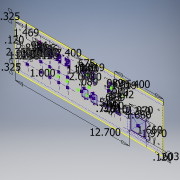
# Autodesk Inventor part: PDU_chassis
Saved by Autodesk Inventor 2017 (Build 210142000, 142)
## iProperties
Created: 2017-02-13
Part Number: PDU_chassis
Material: Generic
Document SubType Name: Modeling
Designer: Zara
Density: 1 g/cm^3
Appearance: Default
Author: Zara
Autodesk Inventor part; units mm, degrees
ref_plane "YZ Plane" through (0, 0, 0) normal (1, 0, 0) x (0, 1, 0)
ref_plane "XZ Plane" through (0, 0, 0) normal (0, 1, 0) x (-1, 0, 0)
ref_plane "XY Plane" through (0, 0, 0) normal (0, 0, 1) x (1, 0, 0)
sketch "Sketch1" plane through (0, 0, 0) normal (0, 0, 1) x (1, 0, 0)
  line L0 (-209.423, -66.294) -> (209.423, -66.294)
  line L1 (209.423, -66.294) -> (209.423, 66.294)
  line L2 (209.423, 66.294) -> (-209.423, 66.294)
  line L3 (-209.423, 66.294) -> (-209.423, -66.294)
  line L4 (-209.423, -66.294) -> (209.423, 66.294) construction
  line L5 (209.423, -66.294) -> (-209.423, 66.294) construction
  point P0 (0, 0)
  dimension "d0" = 418.846
  dimension "d1" = 132.588
  constraints: 12 end point, 2 midpoint, 2 parallel, 1 horizontal, 1 perpendicular
  measures "d0" distance of L1.end L2.end
  measures "d1" distance of L0.end L1.end
extrude "pdu" add sketch "Sketch1" along normal blind 1.651
sketch "dsub9 sketch" plane through (0, 0, 1.651) normal (0, 0, 1) x (1, 0, 0)
  line L0 (206.375, 58.039) -> (-206.375, 58.039) construction
  line L1 (-206.375, 58.039) -> (-206.375, -58.039) construction
  line L2 (-206.375, -58.039) -> (206.375, -58.039) construction
  line L3 (206.375, -58.039) -> (206.375, 58.039) construction
  line L4 (209.423, 66.294) -> (-209.423, 66.294) construction
  line L5 (-209.423, -66.294) -> (209.423, -66.294) construction
  line L6 (-209.423, 66.294) -> (-209.423, -66.294) construction
  line L7 (209.423, -66.294) -> (209.423, 66.294) construction
  arc A0 (-131.445, 36.9951) -> (-133.3231, 38.571) centre (-133.0452, 36.9951) ccw
  arc A1 (-133.3231, 19.3918) -> (-131.445, 20.9677) centre (-133.0452, 20.9677) ccw
  arc A2 (-142.621, 22.374) -> (-141.2987, 20.7981) centre (-141.0208, 22.374) ccw
  arc A3 (-141.2987, 37.1647) -> (-142.621, 35.5888) centre (-141.0208, 35.5888) ccw
  line L8 (-131.445, 36.9951) -> (-131.445, 20.9677)
  line L9 (-142.621, 35.5888) -> (-142.621, 22.374)
  line L10 (-141.2987, 37.1647) -> (-133.3231, 38.571)
  line L11 (-133.3231, 19.3918) -> (-141.2987, 20.7981)
  line L12 (-131.445, 28.9814) -> (-142.621, 28.9814) construction
  line L13 (-137.033, 41.4814) -> (-137.033, 16.4814) construction
  arc A4 (-117.221, 22.374) -> (-115.8987, 20.7981) centre (-115.6208, 22.374) ccw
  arc A5 (-107.9231, 19.3918) -> (-106.045, 20.9677) centre (-107.6452, 20.9677) ccw
  line L14 (-106.045, 28.9814) -> (-117.221, 28.9814) construction
  arc A6 (-115.8987, 37.1647) -> (-117.221, 35.5888) centre (-115.6208, 35.5888) ccw
  line L15 (-115.8987, 37.1647) -> (-107.9231, 38.571)
  line L16 (-106.045, 36.9951) -> (-106.045, 20.9677)
  arc A7 (-106.045, 36.9951) -> (-107.9231, 38.571) centre (-107.6452, 36.9951) ccw
  line L17 (-111.633, 41.4814) -> (-111.633, 16.4814) construction
  line L18 (-107.9231, 19.3918) -> (-115.8987, 20.7981)
  line L19 (-117.221, 35.5888) -> (-117.221, 22.374)
  arc A8 (-91.821, 22.374) -> (-90.4987, 20.7981) centre (-90.2208, 22.374) ccw
  arc A9 (-82.5231, 19.3918) -> (-80.645, 20.9677) centre (-82.2452, 20.9677) ccw
  line L20 (-80.645, 28.9814) -> (-91.821, 28.9814) construction
  arc A10 (-90.4987, 37.1647) -> (-91.821, 35.5888) centre (-90.2208, 35.5888) ccw
  line L21 (-90.4987, 37.1647) -> (-82.5231, 38.571)
  line L22 (-80.645, 36.9951) -> (-80.645, 20.9677)
  arc A11 (-80.645, 36.9951) -> (-82.5231, 38.571) centre (-82.2452, 36.9951) ccw
  line L23 (-86.233, 41.4814) -> (-86.233, 16.4814) construction
  line L24 (-82.5231, 19.3918) -> (-90.4987, 20.7981)
  line L25 (-91.821, 35.5888) -> (-91.821, 22.374)
  arc A12 (-66.421, 22.374) -> (-65.0987, 20.7981) centre (-64.8208, 22.374) ccw
  arc A13 (-57.1231, 19.3918) -> (-55.245, 20.9677) centre (-56.8452, 20.9677) ccw
  line L26 (-55.245, 28.9814) -> (-66.421, 28.9814) construction
  arc A14 (-65.0987, 37.1647) -> (-66.421, 35.5888) centre (-64.8208, 35.5888) ccw
  line L27 (-65.0987, 37.1647) -> (-57.1231, 38.571)
  line L28 (-55.245, 36.9951) -> (-55.245, 20.9677)
  arc A15 (-55.245, 36.9951) -> (-57.1231, 38.571) centre (-56.8452, 36.9951) ccw
  line L29 (-60.833, 41.4814) -> (-60.833, 16.4814) construction
  line L30 (-57.1231, 19.3918) -> (-65.0987, 20.7981)
  line L31 (-66.421, 35.5888) -> (-66.421, 22.374)
  line L32 (-131.445, 32.3846) -> (-131.445, 46.6583) construction
  line L33 (-131.445, 25.0932) -> (-131.445, 19.1695) construction
  line L34 (-135.9942, 38.1) -> (-131.189, 38.9473) construction
  line L35 (-133.9716, 19.5062) -> (-131.2614, 19.0283) construction
  line L36 (-131.445, 24.4508) -> (-131.445, 17.8692) construction
  point P0 (0, 0)
  point P1 (-137.033, 28.9814)
  point P2 (-111.633, 28.9814)
  point P3 (-86.233, 28.9814)
  point P4 (-60.833, 28.9814)
  point P5 (-131.445, 19.0607)
  point P6 (-131.445, 38.9021)
  dimension "d24" = 38.1
  dimension "d13" = 8.255
  dimension "d14" = 8.255
  dimension "d15" = 3.048
  dimension "d16" = 3.048
  dimension "d381" = 3.2004
  dimension "d386" = 3.2004
  dimension "d391" = 3.2004
  dimension "d396" = 3.2004
  dimension "d397" = 16.0274
  dimension "d399" = 11.176
  dimension "d401" = 25
  dimension "d402" = 37.3126
  dimension "d403" = 72.39
  dimension "d406" = 25.4
  dimension "d420" = 100
  dimension "d425" = 19.8415
  constraints: 66 end point, 32 point on circle, 16 centre point, 10 point on line, 8 coincident, 8 tangent, 5 vertical, 4 midpoint, 3 horizontal, 2 parallel, 2 perpendicular, 1 collinear, 86 other
  measures "d13" distance between parallel lines of L4 L0
  measures "d14" distance between parallel lines of L5 L2
  measures "d15" distance between parallel lines of L6 L1
  measures "d16" distance between parallel lines of L7 L3
  measures "d381" diameter of A0
  measures "d386" diameter of A1
  measures "d391" diameter of A2
  measures "d396" diameter of A3
  measures "d397" distance of A1.centre A0.centre
  measures "d399" distance between parallel lines of L9 L8
  measures "d401" distance of L13.start L13.end
  measures "d402" distance between parallel lines of L4 L12
  measures "d403" distance between parallel lines of L13 L6
  measures "d406" distance of A2.centre A4.centre
  measures "d420" angle of L11 L8
  measures "d425" distance of point (-131.445, 38.902) point (-131.445, 19.061)
sketch "CAT7 sketch" plane through (0, 0, 1.651) normal (0, 0, 1) x (1, 0, 0)
  line L0 (-21.463, 40.4114) -> (-4.318, 40.4114)
  line L1 (-4.318, 40.4114) -> (-4.318, 17.5514)
  line L2 (-4.318, 17.5514) -> (-21.463, 17.5514)
  line L3 (-21.463, 17.5514) -> (-21.463, 40.4114)
  line L4 (-29.3489, 28.9814) -> (14.0188, 28.9814) construction
  circle A0 centre (-12.8905, 43.4848) radius 1.1303
  circle A1 centre (-12.8905, 14.478) radius 1.1303
  line L5 (-12.8905, 43.4848) -> (-12.8905, 14.478) construction
  line L6 (-209.423, -66.294) -> (209.423, -66.294) construction
  line L7 (-209.423, 66.294) -> (-209.423, -66.294) construction
  line L8 (32.9446, 29.4386) -> (89.0123, 29.4386) construction
  line L9 (55.7784, 40.4114) -> (71.6026, 40.4114)
  line L10 (72.263, 39.751) -> (72.263, 18.2118)
  line L11 (71.6026, 17.5514) -> (55.7784, 17.5514)
  line L12 (55.118, 18.2118) -> (55.118, 39.751)
  circle A2 centre (63.6905, 43.942) radius 1.1303
  circle A3 centre (63.6905, 14.9352) radius 1.1303
  line L13 (63.6905, 43.942) -> (63.6905, 14.9352) construction
  line L14 (209.423, 66.294) -> (-209.423, 66.294) projected
  line L15 (-209.423, -66.294) -> (209.423, -66.294) projected
  line L16 (209.423, -66.294) -> (209.423, 66.294) projected
  line L17 (209.423, 66.294) -> (-209.423, 66.294) projected
  line L18 (-209.423, 66.294) -> (-209.423, -66.294) projected
  line L19 (3.937, 40.4114) -> (21.082, 40.4114)
  line L20 (21.082, 40.4114) -> (21.082, 17.5514)
  line L21 (21.082, 17.5514) -> (3.937, 17.5514)
  line L22 (3.937, 17.5514) -> (3.937, 40.4114)
  line L23 (12.5095, 43.4848) -> (12.5095, 14.478) construction
  circle A4 centre (12.5095, 43.4848) radius 1.1303
  circle A5 centre (12.5095, 14.478) radius 1.1303
  line L24 (-21.463, -10.3886) -> (-4.318, -10.3886)
  line L25 (-4.318, -10.3886) -> (-4.318, -33.2486)
  line L26 (-4.318, -33.2486) -> (-21.463, -33.2486)
  line L27 (-21.463, -33.2486) -> (-21.463, -10.3886)
  line L28 (-12.8905, -7.3152) -> (-12.8905, -36.322) construction
  circle A6 centre (-12.8905, -7.3152) radius 1.1303
  circle A7 centre (-12.8905, -36.322) radius 1.1303
  line L29 (3.937, -10.3886) -> (21.082, -10.3886)
  line L30 (21.082, -10.3886) -> (21.082, -33.2486)
  line L31 (21.082, -33.2486) -> (3.937, -33.2486)
  line L32 (3.937, -33.2486) -> (3.937, -10.3886)
  line L33 (12.5095, -7.3152) -> (12.5095, -36.322) construction
  circle A8 centre (12.5095, -7.3152) radius 1.1303
  circle A9 centre (12.5095, -36.322) radius 1.1303
  line L34 (-12.8905, -21.8186) -> (115.0098, -21.8186) construction
  arc A10 (72.263, 39.751) -> (71.6026, 40.4114) centre (71.6026, 39.751) ccw
  arc A11 (55.7784, 40.4114) -> (55.118, 39.751) centre (55.7784, 39.751) ccw
  arc A12 (55.118, 18.2118) -> (55.7784, 17.5514) centre (55.7784, 18.2118) ccw
  arc A13 (71.6026, 17.5514) -> (72.263, 18.2118) centre (71.6026, 18.2118) ccw
  point P0 (-21.463, 28.9814)
  point P1 (-12.8905, 40.4114)
  point P2 (-12.8905, 28.9814)
  point P3 (55.118, 40.4114)
  point P4 (72.263, 17.5514)
  point P5 (72.263, 40.4114)
  point P6 (55.118, 17.5514)
  point P7 (55.118, 28.9814)
  point P8 (63.6905, 40.4114)
  point P9 (63.6905, 29.4386)
  point P10 (98.2853, 29.4386)
  point P11 (12.5095, 40.4114)
  point P12 (3.937, 28.9814)
  point P13 (-3.9489, 28.9814)
  point P14 (12.5095, 28.9814)
  point P15 (-12.8905, -10.3886)
  point P16 (-21.463, -21.8186)
  point P17 (-29.3489, -21.8186)
  point P18 (12.5095, -10.3886)
  point P19 (3.937, -21.8186)
  point P20 (-3.9489, -21.8186)
  point P21 (12.5095, -21.8186)
  dimension "d56" = 47.0408
  dimension "d47" = 22.86
  dimension "d49" = 2.2606
  dimension "d50" = 2.2606
  dimension "d51" = 29.0068
  dimension "d146" = 22.86
  dimension "d147" = 17.145
  dimension "d148" = 2.2606
  dimension "d149" = 2.2606
  dimension "d150" = 29.0068
  dimension "d152" = 25.8826
  dimension "d236" = 25.4
  dimension "d239" = 50.8
  dimension "d243" = 137.16
  dimension "d244" = 187.96
  dimension "d245" = 17.145
  dimension "d246" = 25.8826
  dimension "d421" = 0.6604
  constraints: 56 end point, 15 point on line, 14 centre point, 8 point on circle, 8 tangent, 6 midpoint, 5 horizontal, 4 parallel, 4 vertical, 3 equal radius, 2 collinear, 2 perpendicular, 49 other
  measures "d47" distance of L0.end L1.end
  measures "d49" diameter of A0
  measures "d50" diameter of A1
  measures "d51" distance of L5.end L5.start
  measures "d146" distance of point (72.263, 40.411) point (72.263, 17.551)
  measures "d147" distance of point (72.263, 17.551) point (55.118, 17.551)
  measures "d148" diameter of A2
  measures "d149" diameter of A3
  measures "d150" distance of L13.end L13.start
  measures "d152" distance between parallel lines of L14 L9
  measures "d236" distance of L0.start L19.start
  measures "d239" distance of L0.start L24.start
  measures "d243" distance between parallel lines of L16 L10
  measures "d244" distance between parallel lines of L3 L7
  measures "d245" distance of L0.start L0.end
  measures "d246" distance between parallel lines of L17 L0
  measures "d421" radius of A10
sketch "airflow sketch" plane through (0, 0, 1.651) normal (0, 0, 1) x (1, 0, 0)
  line L0 (-209.423, -66.294) -> (209.423, -66.294) construction
  line L1 (113.157, -50.9778) -> (163.195, -50.9778) construction
  line L2 (163.195, -50.9778) -> (163.195, -0.9398) construction
  line L3 (163.195, -0.9398) -> (113.157, -0.9398) construction
  line L4 (113.157, -0.9398) -> (113.157, -50.9778) construction
  line L5 (113.157, -50.9778) -> (163.195, -0.9398) construction
  line L6 (163.195, -50.9778) -> (113.157, -0.9398) construction
  line L7 (-209.423, 66.294) -> (-209.423, -66.294) construction
  line L8 (117.094, -47.0408) -> (159.258, -47.0408)
  line L9 (159.258, -47.0408) -> (159.258, -4.8768)
  line L10 (159.258, -4.8768) -> (117.094, -4.8768)
  line L11 (117.094, -4.8768) -> (117.094, -47.0408)
  line L12 (117.094, -47.0408) -> (159.258, -4.8768) construction
  line L13 (159.258, -47.0408) -> (117.094, -4.8768) construction
  line L14 (108.204, -55.9308) -> (168.148, -55.9308) construction
  line L15 (168.148, -55.9308) -> (168.148, 4.0132) construction
  line L16 (168.148, 4.0132) -> (108.204, 4.0132) construction
  line L17 (108.204, 4.0132) -> (108.204, -55.9308) construction
  line L18 (108.204, -55.9308) -> (168.148, 4.0132) construction
  line L19 (168.148, -55.9308) -> (108.204, 4.0132) construction
  point P0 (0, 0)
  point P1 (0, 0)
  point P2 (138.176, -25.9588)
  point P3 (138.176, -25.9588)
  dimension "d221" = 322.58
  dimension "d222" = 15.3162
  dimension "d223" = 50.038
  dimension "d224" = 50.038
  dimension "d225" = 42.164
  dimension "d226" = 42.164
  dimension "d279" = 59.944
  constraints: 36 end point, 8 midpoint, 6 parallel, 4 coincident, 3 horizontal, 3 perpendicular, 1 point on line
  measures "d221" distance between parallel lines of L4 L7
  measures "d222" distance between parallel lines of L1 L0
  measures "d223" distance of L2.end L3.end
  measures "d224" distance of L1.end L2.end
  measures "d225" distance of L9.end L10.end
  measures "d226" distance of L8.end L9.end
  measures "d279" distance of L15.end L16.end
extrude "airflow cutout" cut sketch "airflow sketch" against normal through all
sketch "sma" plane through (0, 0, 1.651) normal (0, 0, 1) x (1, 0, 0)
  line L0 (-175.133, 2.9121) -> (-175.133, -16.382) construction
  line L1 (-183.1756, -6.223) -> (-164.6712, -6.223) construction
  arc A0 (-177.927, -7.731) -> (-177.927, -4.715) centre (-175.133, -6.223) ccw
  line L2 (-177.927, -4.715) -> (-177.927, -7.731)
  line L3 (-137.033, 41.9354) -> (-137.033, 16.9418) construction
  line L4 (-137.033, 2.9121) -> (-137.033, -16.382) construction
  arc A1 (-139.827, -7.731) -> (-139.827, -4.715) centre (-137.033, -6.223) ccw
  line L5 (-139.827, -4.715) -> (-139.827, -7.731)
  line L6 (-145.0756, -6.223) -> (-126.5712, -6.223) construction
  line L7 (-175.133, -22.4879) -> (-175.133, -41.782) construction
  arc A2 (-177.927, -33.131) -> (-177.927, -30.115) centre (-175.133, -31.623) ccw
  line L8 (-177.927, -30.115) -> (-177.927, -33.131)
  line L9 (-183.1756, -31.623) -> (-164.6712, -31.623) construction
  line L10 (-137.033, -22.4879) -> (-137.033, -41.782) construction
  arc A3 (-139.827, -33.131) -> (-139.827, -30.115) centre (-137.033, -31.623) ccw
  line L11 (-139.827, -30.115) -> (-139.827, -33.131)
  line L12 (-145.0756, -31.623) -> (-126.5712, -31.623) construction
  line L13 (-111.633, -22.4879) -> (-111.633, -41.782) construction
  line L14 (-114.427, -30.115) -> (-114.427, -33.131)
  arc A4 (-114.427, -33.131) -> (-114.427, -30.115) centre (-111.633, -31.623) ccw
  line L15 (-114.427, -4.715) -> (-114.427, -7.731)
  line L16 (-119.6756, -31.623) -> (-101.1712, -31.623) construction
  arc A5 (-114.427, -7.731) -> (-114.427, -4.715) centre (-111.633, -6.223) ccw
  line L17 (-119.6756, -6.223) -> (-101.1712, -6.223) construction
  line L18 (-86.233, -22.4879) -> (-86.233, -41.782) construction
  line L19 (-89.027, -30.115) -> (-89.027, -33.131)
  arc A6 (-89.027, -33.131) -> (-89.027, -30.115) centre (-86.233, -31.623) ccw
  line L20 (-89.027, -4.715) -> (-89.027, -7.731)
  line L21 (-94.2756, -31.623) -> (-75.7712, -31.623) construction
  arc A7 (-89.027, -7.731) -> (-89.027, -4.715) centre (-86.233, -6.223) ccw
  line L22 (-94.2756, -6.223) -> (-75.7712, -6.223) construction
  line L23 (-60.833, -22.4879) -> (-60.833, -41.782) construction
  line L24 (-63.627, -30.115) -> (-63.627, -33.131)
  arc A8 (-63.627, -33.131) -> (-63.627, -30.115) centre (-60.833, -31.623) ccw
  line L25 (-63.627, -4.715) -> (-63.627, -7.731)
  line L26 (-68.8756, -31.623) -> (-50.3712, -31.623) construction
  arc A9 (-63.627, -7.731) -> (-63.627, -4.715) centre (-60.833, -6.223) ccw
  line L27 (-68.8756, -6.223) -> (-50.3712, -6.223) construction
  line L28 (-209.423, 66.294) -> (-209.423, -66.294) projected
  line L29 (-209.423, -66.294) -> (209.423, -66.294) projected
  point P0 (0, 0)
  point P1 (-171.958, -6.223)
  point P2 (-133.858, -6.223)
  point P3 (-171.958, -31.623)
  point P4 (-133.858, -31.623)
  point P5 (-108.458, -31.623)
  point P6 (-111.633, -16.382)
  point P7 (-108.458, -6.223)
  point P8 (-83.058, -31.623)
  point P9 (-86.233, -16.382)
  point P10 (-83.058, -6.223)
  point P11 (-57.658, -31.623)
  point P12 (-60.833, -16.382)
  point P13 (-57.658, -6.223)
  dimension "d123" = 6.35
  dimension "d124" = 5.969
  dimension "d191" = 38.1
  dimension "d198" = 25.4
  dimension "d205" = 25.4
  dimension "d423" = 34.29
  dimension "d424" = 60.071
  constraints: 54 end point, 30 point on circle, 27 point on line, 10 centre point, 3 collinear, 3 horizontal, 3 vertical, 99 other
  measures "d123" diameter of A0
  measures "d124" distance from line of point (-171.958, -6.223) L2
  measures "d191" distance of L0.start L4.start
  measures "d198" distance of L0.start L7.start
  measures "d205" distance of L12.start L16.start
  measures "d423" distance from line of A0.centre L28
  measures "d424" distance from line of A0.centre L29
extrude "sma cutouts" cut sketch "sma" against normal through all
sketch "lc and sc" plane through (0, 0, 1.651) normal (0, 0, 1) x (1, 0, 0)
  arc A0 (-177.927, -7.731) -> (-177.927, -4.715) centre (-175.133, -6.223) ccw projected
  line L0 (-177.927, -7.731) -> (-177.927, -4.715) projected
  line L1 (-209.423, -66.294) -> (209.423, -66.294) projected
  line L2 (209.423, -66.294) -> (209.423, 66.294) projected
  line L3 (209.423, 66.294) -> (-209.423, 66.294) projected
  line L4 (-209.423, 66.294) -> (-209.423, -66.294) projected
  line L5 (63.6905, 43.942) -> (63.6905, 14.9352) construction
  line L6 (55.118, 40.4114) -> (72.263, 40.4114) projected
  line L7 (55.118, 17.5514) -> (55.118, 40.4114) projected
  line L8 (72.263, 17.5514) -> (55.118, 17.5514) projected
  line L9 (72.263, 40.4114) -> (72.263, 17.5514) projected
  circle A1 centre (63.6905, 14.9352) radius 1.1303 projected
  line L10 (-12.8905, -21.8186) -> (115.0098, -21.8186) construction
  line L11 (40.5257, -17.0688) -> (53.5305, -17.0688)
  line L12 (53.5305, -17.0688) -> (53.5305, -26.5684)
  line L13 (53.5305, -26.5684) -> (40.5257, -26.5684)
  line L14 (40.5257, -26.5684) -> (40.5257, -17.0688)
  line L15 (40.5257, -17.0688) -> (53.5305, -26.5684) construction
  line L16 (53.5305, -17.0688) -> (40.5257, -26.5684) construction
  line L17 (38.0111, -21.8186) -> (56.0451, -21.8186) construction
  line L18 (47.0281, -21.8186) -> (47.0281, -14.0945) construction
  line L19 (21.082, -10.3886) -> (21.082, -33.2486) projected
  line L20 (63.6905, 14.9352) -> (63.6905, -41.5551) construction
  line L21 (73.8505, -26.6446) -> (86.9569, -26.6446)
  line L22 (86.9569, -26.6446) -> (86.9569, -16.9926)
  line L23 (86.9569, -16.9926) -> (73.8505, -16.9926)
  line L24 (73.8505, -16.9926) -> (73.8505, -26.6446)
  line L25 (73.8505, -26.6446) -> (86.9569, -16.9926) construction
  line L26 (86.9569, -26.6446) -> (73.8505, -16.9926) construction
  line L27 (71.3867, -21.8186) -> (89.4207, -21.8186) construction
  line L28 (80.4037, -16.3932) -> (80.4037, -27.244) construction
  point P0 (0, 0)
  point P1 (47.0281, -21.8186)
  point P2 (47.0281, -21.8186)
  point P3 (80.4037, -21.8186)
  point P4 (80.4037, -21.8186)
  point P5 (80.4037, -21.8186)
  dimension "d247" = 13.0048
  dimension "d248" = 9.4996
  dimension "d249" = 18.034
  dimension "d262" = 10.16
  dimension "d263" = 18.034
  dimension "d264" = 13.1064
  dimension "d265" = 9.652
  dimension "d266" = 10.16
  constraints: 34 end point, 11 midpoint, 4 coincident, 4 horizontal, 4 parallel, 3 point on line, 2 perpendicular, 2 vertical
  measures "d247" distance of L14.end L12.start
  measures "d248" distance of L12.start L12.end
  measures "d249" distance of L17.start L17.end
  measures "d262" distance between parallel lines of L20 L12
  measures "d263" distance of L27.start L27.end
  measures "d264" distance of L22.end L23.end
  measures "d265" distance of L21.end L22.end
  measures "d266" distance between parallel lines of L20 L24
hole "lc hole" at (56.0451, -21.8186, 1.651) at (38.0111, -21.8186, 1.651) direction (0, 0, -1) diameter 2.3876 end through all clearance for "Countersunk Flat Head Screw ISO 2009/7046" size "M2" standard "ISO"
hole "airflow holes" at (163.195, -0.9398, 1.651) at (113.157, -0.9398, 1.651) at (113.157, -50.9778, 1.651) at (163.195, -50.9778, 1.651) direction (0, 0, -1) diameter 4.4958 end through all clearance for "Flat Head Machine Screw (82)" size "#8" standard "Ansi Unified Screw Threads"
extrude "Extrusion13" cut sketch "CAT7 sketch" against normal blind 25.4 contours L0 L1 L2 L3 | L9 A10 L10 A13 L11 A12 L12 A11 | L19 L20 L21 L22 | L24 L25 L26 L27 | L29 L30 L31 L32
hole "Hole8" at (-12.8905, 43.4848, 1.651) at (-12.8905, 14.478, 1.651) at (12.5095, 43.4848, 1.651) at (12.5095, 14.478, 1.651) at (-12.8905, -7.3152, 1.651) at (-12.8905, -36.322, 1.651) at (12.5095, -7.3152, 1.651) at (12.5095, -36.322, 1.651) at (63.6905, 14.9352, 1.651) at (63.6905, 43.942, 1.651) direction (0, 0, -1) diameter 2.9464 end through all clearance for "Flat Head Machine Screw (82)" size "#4" standard "Ansi Unified Screw Threads"
extrude "Extrusion14" cut sketch "lc and sc" against normal blind 25.4 contours L11 L12 L13 L14 | L24 L23 L22 L21
hole "sc hole" at (89.4207, -21.8186, 1.651) at (71.3867, -21.8186, 1.651) direction (0, 0, -1) diameter 2.4384 end through all clearance for "Flat Head Machine Screw (82)" size "#2" standard "Ansi Unified Screw Threads"
fillet "lc fillets" radius 0.508 4 edges at (40.5257, -26.5684, 0.8255) (53.5305, -17.0688, 0.8255) (53.5305, -26.5684, 0.8255) (40.5257, -17.0688, 0.8255)
fillet "sc fillets" radius 0.508 4 edges at (73.8505, -16.9926, 0.8255) (73.8505, -26.6446, 0.8255) (86.9569, -16.9926, 0.8255) (86.9569, -26.6446, 0.8255)
sketch "brackets" plane through (0, 0, 1.651) normal (0, 0, 1) x (1, 0, 0)
  line L0 (-209.423, 66.294) -> (-209.423, -66.294) construction
  line L1 (-209.423, 54.61) -> (-190.373, 54.61) construction
  line L2 (-190.373, 54.61) -> (-190.373, -54.61) construction
  line L3 (-190.373, -54.61) -> (-209.423, -54.61) construction
  line L4 (-209.423, -54.61) -> (-209.423, 54.61) construction
  line L5 (209.423, 66.294) -> (-209.423, 66.294) construction
  line L6 (209.423, -66.294) -> (209.423, 66.294) construction
  line L7 (209.423, 54.61) -> (190.373, 54.61) construction
  line L8 (190.373, 54.61) -> (190.373, -54.61) construction
  line L9 (190.373, -54.61) -> (209.423, -54.61) construction
  line L10 (209.423, -54.61) -> (209.423, 54.61) construction
  point P0 (0, 0)
  point P1 (196.3674, 41.91)
  point P2 (196.3674, -41.91)
  point P3 (-196.3674, 41.91)
  point P4 (-196.3674, -41.91)
  dimension "d280" = 19.05
  dimension "d281" = 109.22
  dimension "d282" = 11.684
  dimension "d286" = 19.05
  dimension "d287" = 109.22
  dimension "d288" = 11.684
  dimension "d291" = 12.7
  dimension "d292" = 12.7
  dimension "d293" = 12.7
  dimension "d295" = 12.7
  dimension "d297" = 5.9944
  dimension "d298" = 5.9944
  dimension "d306" = 5.9944
  dimension "d307" = 5.9944
  constraints: 16 end point, 4 parallel, 2 horizontal, 2 perpendicular, 2 point on line
  measures "d280" distance of L1.start L1.end
  measures "d281" distance of L1.end L2.end
  measures "d282" distance between parallel lines of L5 L1
  measures "d286" distance of L7.start L7.end
  measures "d287" distance of L7.end L8.end
  measures "d288" distance between parallel lines of L5 L7
  measures "d291" distance from line of point (196.367, -41.91) L9
  measures "d292" distance from line of point (196.367, 41.91) L7
  measures "d293" distance from line of point (-196.367, 41.91) L1
  measures "d295" distance from line of L3 point (-196.367, -41.91)
  measures "d297" distance from line of point (-196.367, 41.91) L2
  measures "d298" distance from line of point (-196.367, -41.91) L2
  measures "d306" distance from line of L8 point (196.367, -41.91)
  measures "d307" distance from line of L8 point (196.367, 41.91)
hole "Hole13" at (-196.3674, 41.91, 1.651) at (-196.3674, -41.91, 1.651) at (196.3674, 41.91, 1.651) at (196.3674, -41.91, 1.651) direction (0, 0, -1) diameter 4.2926 end through all clearance for "Countersunk Flat Head Screw ISO 2009/7046" size "M4" standard "ISO"
extrude "Extrusion16" cut sketch "dsub9 sketch" against normal through all
hole "Hole14" at (-137.033, 41.4814, 1.651) at (-137.033, 16.4814, 1.651) at (-111.633, 41.4814, 1.651) at (-111.633, 16.4814, 1.651) at (-86.233, 41.4814, 1.651) at (-86.233, 16.4814, 1.651) at (-60.833, 41.4814, 1.651) at (-60.833, 16.4814, 1.651) direction (0, 0, -1) diameter 2.9464 end through all
fillet "Fillet4" radius 0.6604 16 edges at (-4.318, 40.4114, 0.8255) (21.082, 40.4114, 0.8255) (-4.318, -10.3886, 0.8255) (21.082, -10.3886, 0.8255) (3.937, 17.5514, 0.8255) (-21.463, 17.5514, 0.8255) (-21.463, -33.2486, 0.8255) (3.937, -33.2486, 0.8255) (-21.463, 40.4114, 0.8255) (3.937, 40.4114, 0.8255) (-21.463, -10.3886, 0.8255) (3.937, -10.3886, 0.8255) (21.082, 17.5514, 0.8255) (21.082, -33.2486, 0.8255) (-4.318, -33.2486, 0.8255) (-4.318, 17.5514, 0.8255)
body "Solid1"
